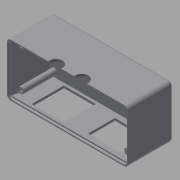
# Autodesk Inventor part: case_top
Saved by Autodesk Inventor 2013 (Build 170138000, 138)
## iProperties
Created: 2014-06-08
Part Number: case_top
Material: Generic
Document SubType Name: Modeling
Designer: Brad
Density: 1 g/cm^3
Author: Brad
Autodesk Inventor part; units mm, degrees
ref_plane "YZ Plane" through (0, 0, 0) normal (1, 0, 0) x (0, 1, 0)
ref_plane "XZ Plane" through (0, 0, 0) normal (0, 1, 0) x (-1, 0, 0)
ref_plane "XY Plane" through (0, 0, 0) normal (0, 0, 1) x (1, 0, 0)
sketch "Sketch1" plane through (0, 0, 0) normal (0, 0, 1) x (1, 0, 0)
  line L0 (-44.45, 18.415) -> (44.45, 18.415)
  line L1 (44.45, 18.415) -> (44.45, -18.415)
  line L2 (44.45, -18.415) -> (-44.45, -18.415)
  line L3 (-44.45, -18.415) -> (-44.45, 18.415)
  line L4 (-46.228, 20.193) -> (46.228, 20.193)
  line L5 (46.228, 20.193) -> (46.228, -20.193)
  line L6 (46.228, -20.193) -> (-46.228, -20.193)
  line L7 (-46.228, -20.193) -> (-46.228, 20.193)
  point P0 (0, 0)
  dimension "d0" = 88.9
  dimension "d2" = 36.83
  dimension "d3" = 1.778
  dimension "d4" = 1.778
  dimension "d5" = 1.778
  dimension "d6" = 1.778
  dimension "d7" = 18.415
  dimension "d8" = 44.45
  constraints: 16 end point, 4 parallel, 2 horizontal, 2 perpendicular
  measures "d0" distance of L0.start L0.end
  measures "d2" distance of L0.end L1.end
  measures "d3" distance between parallel lines of L4 L0
  measures "d4" distance between parallel lines of L5 L1
  measures "d5" distance between parallel lines of L6 L2
  measures "d6" distance between parallel lines of L3 L7
  measures "d7" distance from line of point (0, 0) L0
  measures "d8" distance from line of point (0, 0) L3
extrude "Extrusion1" add sketch "Sketch1" along normal blind 30.48
sketch "Sketch2" plane through (0, 0, 0) normal (0, 0, -1) x (-1, 0, 0)
  line L0 (-46.228, 20.193) -> (46.228, 20.193)
  line L1 (46.228, 20.193) -> (46.228, -20.193)
  line L2 (46.228, -20.193) -> (-46.228, -20.193)
  line L3 (-46.228, -20.193) -> (-46.228, 20.193)
  point P0 (0, 0)
  constraints: 8 end point, 2 parallel, 1 horizontal, 1 perpendicular
extrude "Extrusion2" add sketch "Sketch2" along normal blind 3.81
sketch "Sketch3" plane through (0, 0, 30.48) normal (0, 0, 1) x (1, 0, 0)
  line L0 (44.45, 18.415) -> (44.45, -18.415) projected
  line L1 (44.45, -18.415) -> (-44.45, -18.415) projected
  line L2 (-44.45, -18.415) -> (-44.45, 18.415) projected
  line L3 (-44.45, 18.415) -> (44.45, 18.415)
  line L4 (44.45, 18.415) -> (44.45, -18.415)
  line L5 (44.45, -18.415) -> (-44.45, -18.415)
  line L6 (-44.45, -18.415) -> (-44.45, 18.415)
  line L7 (-45.339, 19.304) -> (45.339, 19.304)
  line L8 (45.339, 19.304) -> (45.339, -19.304)
  line L9 (45.339, -19.304) -> (-45.339, -19.304)
  line L10 (-45.339, -19.304) -> (-45.339, 19.304)
  point P0 (0, 0)
  dimension "d13" = 0.889
  dimension "d15" = 0.889
  dimension "d16" = 0.889
  dimension "d17" = 0.889
  constraints: 16 end point, 4 parallel, 2 horizontal, 2 perpendicular
  measures "d13" distance between parallel lines of L3 L7
  measures "d15" distance between parallel lines of L2 L10
  measures "d16" distance between parallel lines of L8 L0
  measures "d17" distance between parallel lines of L9 L1
extrude "Extrusion3" cut sketch "Sketch3" against normal blind 1.905
sketch "Sketch4" plane through (0, 0, 0) normal (0, 0, 1) x (1, 0, 0)
  line L0 (44.45, 18.415) -> (-44.45, 18.415) projected
  line L1 (-44.45, 18.415) -> (-44.45, -18.415) projected
  line L2 (-44.45, -18.415) -> (44.45, -18.415) projected
  circle A0 centre (-40.64, 14.605) radius 2.3495
  line L3 (-7.0915, 0) -> (0, 0)
  line L4 (0, 0) -> (0, 5.7268)
  circle A1 centre (40.64, 14.605) radius 2.3495
  circle A2 centre (-40.64, -14.605) radius 2.3495
  circle A3 centre (40.64, -14.605) radius 2.3495
  dimension "d20" = 4.699
  dimension "d22" = 3.81
  dimension "d23" = 3.81
  constraints: 4 centre point, 4 end point, 3 symmetric about line, 1 parallel, 1 perpendicular, 3 other
  measures "d20" diameter of A0
  measures "d22" distance from line of L0 A0.centre
  measures "d23" distance from line of L1 A0.centre
extrude "Extrusion4" add sketch "Sketch4" along normal blind 25.4
sketch "Sketch5" plane through (0, 0, 0) normal (0, 0, 1) x (1, 0, 0)
  circle A0 centre (-40.64, 14.605) radius 2.3495 projected
  line L0 (-44.45, -18.415) -> (44.45, -18.415) projected
  circle A1 centre (-40.64, 14.605) radius 1.143
  line L1 (-16.5036, 0) -> (0, 0)
  line L2 (0, 0) -> (0, 9.1282)
  circle A2 centre (40.64, 14.605) radius 1.143
  circle A3 centre (-40.64, -14.605) radius 1.143
  circle A4 centre (40.64, -14.605) radius 1.143
  dimension "d26" = 2.286
  constraints: 4 centre point, 4 end point, 3 symmetric about line, 1 coincident, 1 parallel, 1 perpendicular, 3 other
  measures "d26" diameter of A1
extrude "Extrusion5" cut sketch "Sketch5" along normal blind 25.4 contours A1 | A2 | A3 | A4
sketch "Sketch6" plane through (-44.45, 18.415, 0) normal (0, -1, 0) x (1, 0, 0)
  line L0 (88.9, 28.575) -> (0, 28.575) projected
  line L1 (88.9, 0) -> (88.9, 28.575) projected
  line L2 (44.45, 28.575) -> (44.45, 17.4879)
  circle A0 centre (34.6075, 29.5275) radius 5
  line L3 (-0.889, 28.575) -> (89.789, 28.575) projected
  circle A1 centre (54.2925, 29.5275) radius 5
  line L4 (-1.778, 30.48) -> (90.678, 30.48) projected
  point P0 (44.45, 0)
  dimension "d30" = 44.45
  dimension "d31" = 88.9
  dimension "d32" = 9.8425
  dimension "d34" = 10
  dimension "d37" = 0.9525
  constraints: 2 centre point, 2 end point, 1 midpoint, 1 parallel, 1 symmetric about line, 1 other
  measures "d30" distance between parallel lines of L1 L2
  measures "d31" distance of L0.start L0.end
  measures "d32" distance from line of L2 A0.centre
  measures "d34" diameter of A0
  measures "d37" distance from line of L4 A0.centre
extrude "Extrusion6" cut sketch "Sketch6" against normal blind 5.08 contours A1 L0 | L0 A1 L4 | A1 L4 | A0 L0 | L0 A0 L4 | L4 A0
sketch "Sketch7" plane through (-46.228, -20.193, 30.48) normal (0, -1, 0) x (1, 0, 0)
  line L0 (0, 0) -> (0, -34.29) projected
  line L1 (92.456, -34.29) -> (0, -34.29) projected
  line L2 (55.88, -6.075) -> (82.88, -6.075)
  line L3 (82.88, -6.075) -> (82.88, -26.575)
  line L4 (82.88, -26.575) -> (55.88, -26.575)
  line L5 (55.88, -26.575) -> (55.88, -6.075)
  line L6 (14.9026, -4.075) -> (39.4026, -4.075)
  line L7 (39.4026, -4.075) -> (39.4026, -28.575)
  line L8 (39.4026, -28.575) -> (14.9026, -28.575)
  line L9 (14.9026, -28.575) -> (14.9026, -4.075)
  line L10 (48.26, -34.29) -> (48.26, -15.4133)
  line L11 (0, 0) -> (92.456, 0) projected
  line L12 (69.38, -26.575) -> (69.38, -17.756)
  line L13 (27.1526, -28.575) -> (27.1526, -15.4133)
  point P0 (46.228, -30.48)
  dimension "d38" = 27
  dimension "d41" = 20.5
  dimension "d42" = 24.5
  dimension "d43" = 24.5
  dimension "d44" = 92.456
  dimension "d45" = 48.26
  dimension "d48" = 2
  dimension "d49" = 5.715
  dimension "d68" = 7.62
  dimension "d69" = 13.5
  dimension "d70" = 21.12
  dimension "d71" = 12.25
  dimension "d72" = 21.1074
  constraints: 22 end point, 6 parallel, 3 perpendicular, 2 horizontal, 2 midpoint, 1 point on line
  measures "d38" distance of L2.start L2.end
  measures "d41" distance of L2.end L3.end
  measures "d42" distance of L6.start L6.end
  measures "d43" distance of L6.end L7.end
  measures "d44" distance of L1.start L0.end
  measures "d45" distance between parallel lines of L0 L10
  measures "d48" distance between parallel lines of L6 L2
  measures "d49" distance between parallel lines of L1 L8
  measures "d68" distance between parallel lines of L5 L10
  measures "d69" distance between parallel lines of L12 L5
  measures "d70" distance between parallel lines of L12 L10
  measures "d71" distance between parallel lines of L7 L13
  measures "d72" distance between parallel lines of L10 L13
extrude "Extrusion7" cut sketch "Sketch7" against normal blind 5.08
sketch "Sketch9" plane through (0, 0, 0) normal (0, 0, 1) x (1, 0, 0)
  circle A0 centre (-40.64, 14.605) radius 2.3495 projected
  line L0 (44.45, 18.415) -> (-44.45, 18.415) projected
  line L1 (-44.45, 18.415) -> (-44.45, -18.415) projected
  arc A1 (-41.9028, 16.5863) -> (-42.6213, 15.8678) centre (-40.64, 14.605) ccw
  line L2 (-44.45, 18.415) -> (-44.45, 18.415)
  line L3 (-44.45, 18.415) -> (-44.45, 18.415)
  line L4 (-43.7316, 18.415) -> (-41.9028, 16.5863)
  line L5 (-44.45, 17.6966) -> (-42.6213, 15.8678)
  line L6 (-44.45, 18.415) -> (-42.9203, 16.8853)
  line L7 (-44.45, 17.6966) -> (-44.45, 18.415)
  line L8 (-44.45, 18.415) -> (-43.7316, 18.415)
  line L9 (-12.1408, 0) -> (0, 0)
  line L10 (0, 0) -> (0, 7.1556)
  arc A2 (42.6213, 15.8678) -> (41.9028, 16.5863) centre (40.64, 14.605) ccw
  line L11 (44.45, 18.415) -> (44.45, 18.415)
  line L12 (44.45, 18.415) -> (44.45, 18.415)
  line L13 (43.7316, 18.415) -> (41.9028, 16.5863)
  line L14 (44.45, 17.6966) -> (42.6213, 15.8678)
  line L15 (44.45, 17.6966) -> (44.45, 18.415)
  line L16 (44.45, 18.415) -> (43.7316, 18.415)
  arc A3 (-42.6213, -15.8678) -> (-41.9028, -16.5863) centre (-40.64, -14.605) ccw
  line L17 (-43.7316, -18.415) -> (-41.9028, -16.5863)
  line L18 (-44.45, -17.6966) -> (-42.6213, -15.8678)
  line L19 (-44.45, -17.6966) -> (-44.45, -18.415)
  line L20 (-44.45, -18.415) -> (-43.7316, -18.415)
  arc A4 (41.9028, -16.5863) -> (42.6213, -15.8678) centre (40.64, -14.605) ccw
  line L21 (44.45, -17.6966) -> (42.6213, -15.8678)
  line L22 (43.7316, -18.415) -> (41.9028, -16.5863)
  line L23 (44.45, -17.6966) -> (44.45, -18.415)
  line L24 (44.45, -18.415) -> (43.7316, -18.415)
  point P0 (44.45, -18.415)
  point P1 (-44.45, -18.415)
  point P2 (44.45, -18.415)
  dimension "d56" = 45
  dimension "d57" = 45
  dimension "d58" = 0.508
  dimension "d60" = 0.508
  constraints: 46 end point, 25 symmetric about line, 10 point on circle, 6 point on line, 4 centre point, 2 parallel, 1 coincident, 1 collinear, 1 concentric, 1 perpendicular, 3 other
  measures "d56" angle of L3 L5
  measures "d57" angle of L0 L4
  measures "d58" distance between parallel lines of L6 L4
  measures "d60" distance between parallel lines of L6 L5
extrude "Extrusion8" add sketch "Sketch9" along normal blind 25.4 contours A0 L5 L1 L0 L4 | L15 L14 A2 L13 L0 | L18 A3 L17 L20 L1 | A4 L21 L23 L24 L22
fillet "Fillet1" radius 3.175 8 edges at (-46.228, -20.193, 13.335) (46.228, -20.193, 13.335) (46.228, 20.193, 13.335) (-46.228, 20.193, 13.335) (45.339, 19.304, 29.5275) (45.339, -19.304, 29.5275) (-45.339, -19.304, 29.5275) (-45.339, 19.304, 29.5275)
fillet "Fillet2" radius 1.778 8 edges at (-45.2981, -19.2631, -3.81) (-46.228, 0, -3.81) (-45.2981, 19.2631, -3.81) (0, 20.193, -3.81) (45.2981, 19.2631, -3.81) (46.228, 0, -3.81) (45.2981, -19.2631, -3.81) (0, -20.193, -3.81)
body "Solid1"
